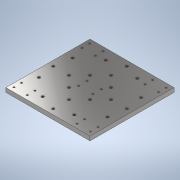
# Autodesk Inventor part: Mesa
Saved by Autodesk Inventor 2020 (Build 240168000, 168)
## iProperties
Created: 2020-05-08
Part Number: Mesa
Material: Steel, Mild
Document SubType Name: Modeling
Designer: Pipi
Density: 7.85 g/cm^3
Appearance: Semi-Polished
Mass: 3081.59 g
Surface Area: 994.228 cm^2
Volume: 392.56 cm^3
Author: Pipi
Autodesk Inventor part; units mm, degrees
ref_plane "YZ Plane" through (0, 0, 0) normal (1, 0, 0) x (0, 1, 0)
ref_plane "XZ Plane" through (0, 0, 0) normal (0, 1, 0) x (-1, 0, 0)
ref_plane "XY Plane" through (0, 0, 0) normal (0, 0, 1) x (1, 0, 0)
sketch "Boceto1" plane through (0, 0, 0) normal (0, 1, 0) x (-1, 0, 0)
  line L0 (0, 0) -> (200, 0)
  line L1 (200, 0) -> (200, -200)
  line L2 (200, -200) -> (0, -200)
  line L3 (0, 0) -> (0, -200)
  line L4 (175, -50) -> (175, -150)
  line L5 (175, -150) -> (25, -150)
  line L6 (25, -150) -> (25, -50)
  line L7 (25, -50) -> (175, -50)
  line L8 (50, -175) -> (50, -25)
  line L9 (150, -175) -> (50, -175)
  line L10 (150, -25) -> (150, -175)
  line L11 (50, -25) -> (150, -25)
  circle A0 centre (75, -75) radius 3
  circle A1 centre (125, -75) radius 3
  circle A2 centre (75, -125) radius 3
  circle A3 centre (125, -125) radius 3
  line L12 (155, -5) -> (195, -5)
  circle A4 centre (100, -12.5) radius 3
  circle A5 centre (100, -187.5) radius 3
  circle A6 centre (12.5, -100) radius 3
  circle A7 centre (187.5, -100) radius 3
  circle A8 centre (50, -100) radius 3
  circle A9 centre (150, -100) radius 3
  circle A10 centre (100, -150) radius 3
  circle A11 centre (100, -50) radius 3
  circle A12 centre (62.5, -25) radius 3
  circle A13 centre (137.5, -25) radius 3
  circle A14 centre (62.5, -175) radius 3
  circle A15 centre (137.5, -175) radius 3
  line L13 (155, -5) -> (155, -33)
  line L14 (155, -33) -> (195, -33)
  line L15 (195, -33) -> (195, -5)
  line L16 (187.5, -100) -> (187.5, -60)
  line L17 (187.5, -60) -> (187.5, -140)
  line L18 (187.5, -140) -> (181.5, -140)
  line L19 (181.5, -140) -> (181.5, -60)
  line L20 (181.5, -60) -> (187.5, -60)
  line L21 (12.5, -100) -> (12.5, -140)
  line L22 (12.5, -140) -> (12.5, -60)
  line L23 (12.5, -60) -> (18.5, -60)
  line L24 (18.5, -60) -> (18.5, -140)
  line L25 (18.5, -140) -> (12.5, -140)
  circle A16 centre (181.5, -60) radius 3
  circle A17 centre (181.5, -140) radius 3
  circle A18 centre (18.5, -140) radius 3
  circle A19 centre (18.5, -60) radius 3
  line L26 (100, -100) -> (100, -105)
  line L27 (100, -105) -> (100, -95)
  line L28 (100, -95) -> (100, -100)
  line L29 (100, -100) -> (95, -100)
  line L30 (95, -100) -> (105, -100)
  line L31 (100, -100) -> (80, -100)
  line L32 (80, -100) -> (121, -100)
  line L33 (121, -100) -> (121, -120)
  line L34 (121, -120) -> (121, -80)
  line L35 (121, -80) -> (79, -80)
  line L36 (79, -80) -> (79, -120)
  line L37 (79, -120) -> (121, -120)
  line L38 (79, -80) -> (83, -80)
  line L39 (83, -80) -> (83, -120)
  line L40 (121, -120) -> (117, -120)
  line L41 (117, -120) -> (117, -80)
  line L42 (83, -80) -> (83, -90)
  line L43 (83, -90) -> (117, -90)
  line L44 (83, -120) -> (83, -110)
  line L45 (83, -110) -> (117, -110)
  circle A20 centre (83, -90) radius 2
  circle A21 centre (83, -110) radius 2
  circle A22 centre (117, -110) radius 2
  circle A23 centre (117, -90) radius 2
  line L46 (195, -5) -> (191, -5)
  line L47 (191, -5) -> (191, -33)
  line L48 (155, -5) -> (159, -5)
  line L49 (159, -5) -> (159, -33)
  line L50 (159, -5) -> (159, -10)
  line L51 (159, -33) -> (159, -28)
  line L52 (159, -28) -> (191, -28)
  line L53 (159, -10) -> (191, -10)
  circle A24 centre (191, -10) radius 2
  circle A25 centre (159, -10) radius 2
  circle A26 centre (159, -28) radius 2
  circle A27 centre (191, -28) radius 2
  line L54 (45, -5) -> (5, -5)
  line L55 (45, -5) -> (45, -33)
  line L56 (45, -33) -> (5, -33)
  line L57 (5, -33) -> (5, -5)
  line L58 (5, -5) -> (9, -5)
  line L59 (9, -5) -> (9, -33)
  line L60 (45, -5) -> (41, -5)
  line L61 (41, -5) -> (41, -33)
  line L62 (41, -5) -> (41, -10)
  line L63 (41, -33) -> (41, -28)
  line L64 (41, -28) -> (9, -28)
  line L65 (41, -10) -> (9, -10)
  circle A28 centre (9, -10) radius 2
  circle A29 centre (41, -10) radius 2
  circle A30 centre (41, -28) radius 2
  circle A31 centre (9, -28) radius 2
  line L66 (155, -195) -> (195, -195)
  line L67 (155, -195) -> (155, -167)
  line L68 (155, -167) -> (195, -167)
  line L69 (195, -167) -> (195, -195)
  line L70 (195, -195) -> (191, -195)
  line L71 (191, -195) -> (191, -167)
  line L72 (155, -195) -> (159, -195)
  line L73 (159, -195) -> (159, -167)
  line L74 (159, -195) -> (159, -190)
  line L75 (159, -167) -> (159, -172)
  line L76 (159, -172) -> (191, -172)
  line L77 (159, -190) -> (191, -190)
  circle A32 centre (191, -190) radius 2
  circle A33 centre (159, -190) radius 2
  circle A34 centre (159, -172) radius 2
  circle A35 centre (191, -172) radius 2
  line L78 (0, -100) -> (7, -100)
  line L79 (45, -195) -> (5, -195)
  line L80 (45, -195) -> (45, -167)
  circle A36 centre (41, -172) radius 2
  line L81 (45, -167) -> (5, -167)
  line L82 (5, -167) -> (5, -195)
  line L83 (41, -167) -> (41, -172)
  circle A37 centre (41, -190) radius 2
  line L84 (41, -195) -> (41, -167)
  line L85 (41, -195) -> (41, -190)
  line L86 (41, -172) -> (9, -172)
  circle A38 centre (9, -172) radius 2
  line L87 (41, -190) -> (9, -190)
  line L88 (9, -195) -> (9, -167)
  circle A39 centre (9, -190) radius 2
  line L89 (5, -195) -> (9, -195)
  line L90 (45, -195) -> (41, -195)
  circle A40 centre (150, -100) radius 14
  circle A41 centre (125, -75) radius 14
  circle A42 centre (100, -50) radius 14
  circle A43 centre (137.5, -25) radius 14
  circle A44 centre (100, -12.5) radius 14
  circle A45 centre (62.5, -25) radius 14
  circle A46 centre (18.5, -60) radius 14
  circle A47 centre (50, -100) radius 14
  circle A48 centre (75, -75) radius 14
  circle A49 centre (75, -125) radius 14
  circle A50 centre (100, -150) radius 14
  circle A51 centre (125, -125) radius 14
  circle A52 centre (181.5, -140) radius 14
  circle A53 centre (187.5, -100) radius 14
  circle A54 centre (181.5, -60) radius 14
  circle A55 centre (137.5, -175) radius 14
  circle A56 centre (100, -187.5) radius 14
  circle A57 centre (62.5, -175) radius 14
  circle A58 centre (18.5, -140) radius 14
  circle A59 centre (12.5, -100) radius 14
  circle A60 centre (150, -150) radius 3
  circle A61 centre (50, -150) radius 3
  circle A62 centre (150, -50) radius 3
  circle A63 centre (50, -50) radius 3
  dimension "d0" = 200
  dimension "d1" = 200
  dimension "d2" = 200
  dimension "d6" = 100
  dimension "d7" = 150
  dimension "d8" = 100
  dimension "d11" = 6
  dimension "d14" = 6
  dimension "d15" = 6
  dimension "d16" = 12.5
  dimension "d17" = 6
  dimension "d18" = 6
  dimension "d19" = 6
  dimension "d20" = 6
  dimension "d21" = 12.5
  dimension "d26" = 50
  dimension "d27" = 50
  dimension "d30" = 28
  dimension "d51" = 40
  dimension "d52" = 80
  dimension "d53" = 6
  dimension "d54" = 40
  dimension "d55" = 80
  dimension "d56" = 6
  dimension "d57" = 6
  dimension "d58" = 6
  dimension "d59" = 6
  dimension "d60" = 6
  dimension "d98" = 4
  dimension "d99" = 4
  dimension "d100" = 10
  dimension "d101" = 10
  dimension "d102" = 4
  dimension "d103" = 4
  dimension "d104" = 4
  dimension "d105" = 4
  dimension "d116" = 4
  dimension "d117" = 4
  dimension "d118" = 5
  dimension "d119" = 5
  dimension "d120" = 4
  dimension "d121" = 4
  dimension "d122" = 4
  dimension "d123" = 4
  dimension "d124" = 5
  dimension "d166" = 20
  dimension "d167" = 20
  dimension "d236" = 21
  dimension "d237" = 100
  dimension "d238" = 21
  dimension "d240" = 28
  dimension "d241" = 28
  dimension "d242" = 28
  dimension "d243" = 28
  dimension "d244" = 28
  dimension "d245" = 28
  dimension "d246" = 28
  dimension "d247" = 28
  dimension "d248" = 28
  dimension "d249" = 28
  dimension "d250" = 28
  dimension "d251" = 28
  dimension "d252" = 28
  dimension "d253" = 28
  constraints: 182 end point, 64 centre point, 58 point on line, 43 coincident, 23 perpendicular, 16 symmetric about line, 4 midpoint, 3 horizontal, 3 vertical, 1 collinear, 1 parallel, 4 other
  measures "d0" distance of L0.start L0.end
  measures "d1" distance of L0.end L1.end
  measures "d2" distance of L1.end L2.end
  measures "d6" distance of L7.end L4.end
  measures "d7" distance of L4.end L6.start
  measures "d8" distance of L11.start L11.end
  measures "d11" diameter of A0
  measures "d14" diameter of A4
  measures "d15" diameter of A6
  measures "d16" distance from line of L1 L16.start
  measures "d17" diameter of A8
  measures "d18" diameter of A10
  measures "d19" diameter of A11
  measures "d20" diameter of A12
  measures "d21" horizontal distance of A0.centre A12.centre
  measures "d26" distance of A1.centre A3.centre
  measures "d27" distance of A2.centre A3.centre
  measures "d30" distance of L12.start L13.end
  measures "d51" distance of L16.start L16.end
  measures "d52" distance of L16.end L17.end
  measures "d53" distance of L17.end L18.end
  measures "d54" distance of L21.start L21.end
  measures "d55" distance of L21.end L22.end
  measures "d56" distance of L22.end L23.end
  measures "d57" diameter of A16
  measures "d58" diameter of A17
  measures "d59" diameter of A18
  measures "d60" diameter of A19
  measures "d98" distance of L35.end L38.end
  measures "d99" distance of L33.end L40.end
  measures "d100" distance of L38.end L42.end
  measures "d101" distance of L39.end L44.end
  measures "d102" diameter of A20
  measures "d103" diameter of A21
  measures "d104" diameter of A22
  measures "d105" diameter of A23
  measures "d116" distance of L12.end L46.end
  measures "d117" distance of L12.start L48.end
  measures "d118" distance of L48.end L50.end
  measures "d119" distance of L49.end L51.end
  measures "d120" diameter of A24
  measures "d121" diameter of A25
  measures "d122" diameter of A26
  measures "d123" diameter of A27
  measures "d124" distance between parallel lines of L0 L12
  measures "d166" distance from line of L35 L26.start
  measures "d167" distance between parallel lines of L37 L30
  measures "d236" distance from line of L36 L26.start
  measures "d237" distance from line of L3 L26.start
  measures "d238" distance between parallel lines of L26 L34
  measures "d240" diameter of A40
  measures "d241" diameter of A41
  measures "d242" diameter of A42
  measures "d243" diameter of A43
  measures "d244" diameter of A44
  measures "d245" diameter of A45
  measures "d246" diameter of A46
  measures "d247" diameter of A47
  measures "d248" diameter of A48
  measures "d249" diameter of A49
  measures "d250" diameter of A50
  measures "d251" diameter of A51
  measures "d252" diameter of A52
  measures "d253" diameter of A53
extrude "Extrusión1" add sketch "Boceto1" along normal blind 10 contours L0 A44 L11 A45 L8 A63 L7 A46 L22 A59 L3 | L0 A44 L11 | A59 L22 A6 L21 L3 | L0 L1 A53 L16 A54 L7 A62 L10 A43 L11 A44 | A44 L11 A43 L10 A62 L7 A42 A63 L8 A45 | L11 A44 | A59 L24 L21 A6 L22 | L22 A46 L24 A59 | A59 L21 A58 L5 A61 L8 A57 L9 A56 L2 L3 | A45 L8 L11 A12 | L11 A12 L8 A45 | A46 L7 L6 L24 A19 L23 L22 | L22 L23 A19 L24 A46 | A59 L6 L24 | L24 A46 L6 A59 | A59 L24 A58 L21 | L1 A53 L17 A7 L16 | A43 L10 L11 A13 | L11 A13 L10 A43 | A46 L6 L7 | L7 A63 L8 A47 A61 L5 A58 L6 A59 A46 | A59 L6 A58 L24 | A59 L6 | A56 L9 L2 | A58 L24 A18 L25 L21 | L21 L25 A18 L24 A58 L6 L5 | L1 L2 A56 L9 A55 L10 A60 L5 A52 L17 A53 | A53 L19 A54 L16 | L16 A7 L17 A53 L19 | A63 L7 L8 | L8 L7 A63 | L7 L8 A63 | A56 L9 | L9 A57 L8 A61 L5 A50 A60 L10 A55 A56 | L5 L6 A58 | L17 A52 L19 A53 | A54 L19 A16 L20 L16 | L16 L20 A16 L19 A54 L4 L7 | A53 L4 A54 L19 | L19 A53 L4 | L7 A63 L8 | L7 A42 A62 L10 A40 A60 L5 A50 A61 L8 A47 A63 | A62 L7 L10 | L10 L7 A62 | A57 L8 L9 A14 | L9 A14 L8 A57 | A61 L8 L5 | L5 L8 A61 | A52 L5 L4 L19 A17 L18 L17 | L17 L18 A17 L19 A52 | L19 A52 L4 A53 | A53 L4 A52 L5 A60 L10 A40 A62 L7 A54 | L4 A53 | A42 L7 A11 | L7 A11 A42 | L10 A62 L7 | L7 A62 L10 | A47 L8 A8 | L8 A8 A47 | A55 L10 L9 A15 | L9 A15 L10 A55 | L8 A61 L5 | L5 A61 L8 | A54 L7 L4 | A52 L4 L5 | A40 L10 A9 | L10 A9 A40 | A60 L5 L10 | L10 L5 A60 | A50 L5 A10 | L5 A10 A50 | L5 L10 A60 | L5 A60 L10 | L12 L49 A25 A26 L14 L13 | L12 L47 A24 L53 A25 L49 | L12 L15 L14 L47 A27 A24 | A25 L53 L49 | L49 A25 | L49 A26 L52 A27 L47 L14 | A24 L47 | L47 L53 A24 | L53 A25 L49 | L53 A24 L47 A27 L52 A26 L49 A25 | A26 L49 | L49 L52 A26 | L47 A24 L53 | A26 L52 L49 | A27 L52 L47 | L47 A27 | L52 A27 L47 | L30 L32 L41 A22 L45 A21 L39 L31 L29 | L29 L31 L39 A20 L43 A23 L41 L32 L30 | L39 A21 A49 L36 A48 A20 | L41 A23 A41 L34 L32 | L32 L33 A51 L41 A22 | A20 L39 | L39 L43 A20 | A21 L45 L39 | L39 A21 | A22 L41 | L41 L45 A22 | A23 L43 L41 | L41 A23 | L39 A20 L43 | L39 A48 L35 A41 L41 A23 L43 A20 | L45 A21 L39 | L45 A22 L41 A51 L37 A49 L39 A21 | A51 L37 L33 | L33 L37 L41 A51 | A41 L41 L35 L34 | L34 L35 A41 | L41 A22 L45 | L43 A23 L41 | A48 L36 L35 L39 | L39 L35 A48 | A49 L37 L39 | L39 L37 L36 A49 | L41 L37 A51 | A41 L35 L41 | L35 L36 A48 | L37 A49 L36 | L55 L56 L61 A30 A29 L54 | L61 A29 L65 A28 L59 L54 | L59 A28 A31 L56 L57 L54 | A29 L61 | L61 L65 A29 | L56 L59 A31 L64 A30 L61 | A28 L65 L59 | L59 A28 | L61 A29 L65 | A29 L61 A30 L64 A31 L59 A28 L65 | A30 L64 L61 | L61 A30 | L65 A28 L59 | A31 L59 | L59 L64 A31 | L64 A30 L61 | A31 L64 L59 | L67 L68 L73 A34 A33 L66 | L73 A33 L77 A32 L71 L66 | L71 A32 A35 L68 L69 L66 | A33 L73 | L73 L77 A33 | L68 L71 A35 L76 A34 L73 | A32 L77 L71 | L71 A32 | L73 A33 L77 | L73 A34 L76 A35 L71 A32 L77 A33 | A34 L76 L73 | L73 A34 | L77 A32 L71 | L73 L76 A34 | A35 L71 | L71 L76 A35 | L71 A35 L76 | L79 L84 A37 A36 L83 L81 L80 | L79 L88 A39 L87 A37 L84 | L79 L82 L81 L88 A38 A39 | L84 A37 | A37 L87 L84 | L83 A36 L86 A38 L88 L81 | A39 L88 | L88 L87 A39 | L87 A39 L88 A38 L86 A36 L84 A37 | A37 L84 L87 | L83 L86 A36 | A36 L84 L83 | L88 A39 L87 | L88 A38 | A38 L86 L88 | L86 L84 A36 | L88 L86 A38
hole "Agujero1" at (-9, 0, -10) at (-9, 0, -28) at (-41, 0, -28) at (-41, 0, -10) at (-9, 0, -172) at (-9, 0, -190) at (-41, 0, -190) at (-41, 0, -172) at (-159, 0, -190) at (-159, 0, -172) at (-191, 0, -172) at (-191, 0, -190) at (-159, 0, -28) at (-159, 0, -10) at (-191, 0, -10) at (-191, 0, -28) direction (0, 1, 0) diameter 4 depth 12 tip angle 118
thread "Rosca6" size "M4x0.7" class "6H" standard "ISO Metric profile" length 430
thread "Rosca7" size "M4x0.7" class "6H" standard "ISO Metric profile" length 430
thread "Rosca8" size "M4x0.7" class "6H" standard "ISO Metric profile" length 430
thread "Rosca9" size "M4x0.7" class "6H" standard "ISO Metric profile" length 430
thread "Rosca10" size "M4x0.7" class "6H" standard "ISO Metric profile" length 430
thread "Rosca11" size "M4x0.7" class "6H" standard "ISO Metric profile" length 430
thread "Rosca12" size "M4x0.7" class "6H" standard "ISO Metric profile" length 430
thread "Rosca13" size "M4x0.7" class "6H" standard "ISO Metric profile" length 430
thread "Rosca14" size "M4x0.7" class "6H" standard "ISO Metric profile" length 430
thread "Rosca15" size "M4x0.7" class "6H" standard "ISO Metric profile" length 430
thread "Rosca16" size "M4x0.7" class "6H" standard "ISO Metric profile" length 430
thread "Rosca17" size "M4x0.7" class "6H" standard "ISO Metric profile" length 430
thread "Rosca18" size "M4x0.7" class "6H" standard "ISO Metric profile" length 430
thread "Rosca19" size "M4x0.7" class "6H" standard "ISO Metric profile" length 430
thread "Rosca20" size "M4x0.7" class "6H" standard "ISO Metric profile" length 430
thread "Rosca21" size "M4x0.7" class "6H" standard "ISO Metric profile" length 430
thread "Thread22" size "M6x1" class "6H" standard "ANSI Metric M Profile" length 40
thread "Thread23" size "M6x1" class "6H" standard "ANSI Metric M Profile" length 40
thread "Thread24" size "M6x1" class "6H" standard "ANSI Metric M Profile" length 40
thread "Thread25" size "M6x1" class "6H" standard "ANSI Metric M Profile" length 40
thread "Thread26" size "M6x1" class "6H" standard "ANSI Metric M Profile" length 40
thread "Thread27" size "M6x1" class "6H" standard "ANSI Metric M Profile" length 40
thread "Thread28" size "M6x1" class "6H" standard "ANSI Metric M Profile" length 40
thread "Thread29" size "M6x1" class "6H" standard "ANSI Metric M Profile" length 40
thread "Thread30" size "M6x1" class "6H" standard "ANSI Metric M Profile" length 40
thread "Thread31" size "M6x1" class "6H" standard "ANSI Metric M Profile" length 40
thread "Thread32" size "M6x1" class "6H" standard "ANSI Metric M Profile" length 40
thread "Thread33" size "M6x1" class "6H" standard "ANSI Metric M Profile" length 40
thread "Thread34" size "M6x1" class "6H" standard "ANSI Metric M Profile" length 40
thread "Thread35" size "M6x1" class "6H" standard "ANSI Metric M Profile" length 40
thread "Thread36" size "M6x1" class "6H" standard "ANSI Metric M Profile" length 40
thread "Thread37" size "M6x1" class "6H" standard "ANSI Metric M Profile" length 40
thread "Thread38" size "M6x1" class "6H" standard "ANSI Metric M Profile" length 40
thread "Thread39" size "M6x1" class "6H" standard "ANSI Metric M Profile" length 40
thread "Thread40" size "M6x1" class "6H" standard "ANSI Metric M Profile" length 40
thread "Thread41" size "M6x1" class "6H" standard "ANSI Metric M Profile" length 40
hole "Agujero2" at (-117, 0, -90) at (-83, 0, -90) at (-117, 0, -110) at (-83, 0, -110) direction (0, 1, 0) diameter 4 depth 12 tip angle 118
thread "Rosca42" size "M4x0.7" class "6H" standard "ISO Metric profile" length 430
thread "Rosca43" size "M4x0.7" class "6H" standard "ISO Metric profile" length 430
thread "Rosca44" size "M4x0.7" class "6H" standard "ISO Metric profile" length 430
thread "Rosca45" size "M4x0.7" class "6H" standard "ISO Metric profile" length 430
